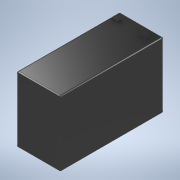
# Autodesk Inventor part: battery
Saved by Autodesk Inventor 2021 (Build 250183000, 183)
## iProperties
Created: 2021-03-02
Part Number: battery
Material: Generic
Document SubType Name: Modeling
Designer: Mateusz
Density: 1 g/cm^3
Appearance: Default
Author: Mateusz
Autodesk Inventor part; units mm, degrees
ref_plane "YZ Plane" through (0, 0, 0) normal (1, 0, 0) x (0, 1, 0)
ref_plane "XZ Plane" through (0, 0, 0) normal (0, 1, 0) x (-1, 0, 0)
ref_plane "XY Plane" through (0, 0, 0) normal (0, 0, 1) x (1, 0, 0)
sketch "Sketch1" plane through (0, 0, 0) normal (0, 1, 0) x (-1, 0, 0)
  line L0 (0, 0) -> (0, -148)
  line L1 (0, -148) -> (63, -148)
  line L2 (63, -148) -> (63, 0)
  line L3 (63, 0) -> (0, 0)
  dimension "d0" = 148
  dimension "d1" = 63
  constraints: 8 end point, 3 perpendicular, 1 vertical
  measures "d0" distance of L0.start L0.end
  measures "d1" distance of L0.end L1.end
extrude "Extrusion1" add sketch "Sketch1" along normal blind 94
sketch "Sketch2" plane through (0, 94, 0) normal (0, 1, 0) x (1, 0, 0)
  line L0 (0, 148) -> (-63, 148) projected
  line L1 (-63, 148) -> (-63, 136)
  line L2 (-63, 148) -> (-63, 0) projected
  line L3 (-63, 136) -> (-55, 136)
  line L4 (-55, 136) -> (-48, 136)
  line L5 (-48, 136) -> (-48, 134)
  line L6 (-48, 134) -> (-55, 134)
  line L7 (-55, 134) -> (-55, 136)
  line L8 (0, 0) -> (0, 148) projected
  line L9 (0, 148) -> (0, 136)
  line L10 (0, 136) -> (-8, 136)
  line L11 (-8, 136) -> (-8, 134)
  line L12 (-8, 134) -> (-15, 134)
  line L13 (-15, 134) -> (-15, 136)
  line L14 (-15, 136) -> (-8, 136)
  dimension "d4" = 12
  dimension "d5" = 8
  dimension "d6" = 7
  dimension "d7" = 2
  dimension "d8" = 12
  dimension "d9" = 8
  dimension "d10" = 2
  dimension "d11" = 7
  constraints: 24 end point, 7 point on line, 5 perpendicular
  measures "d4" distance of L0.end L1.end
  measures "d5" distance of L1.end L3.end
  measures "d6" distance of L3.end L4.end
  measures "d7" distance of L4.end L5.end
  measures "d8" distance of L0.start L9.end
  measures "d9" distance of L9.end L10.end
  measures "d10" distance of L10.end L11.end
  measures "d11" distance of L11.end L12.end
extrude "Extrusion2" add sketch "Sketch2" along normal blind 5
sketch "Sketch3" plane through (-55, 94, -134) normal (0, 0, 1) x (1, 0, 0)
  line L0 (0, 5) -> (7, 5) projected
  line L1 (0, 5) -> (0, 3)
  line L2 (0, 0) -> (0, 5) projected
  line L3 (0, 3) -> (7, 3)
  line L4 (7, 0) -> (7, 5) projected
  line L5 (7, 5) -> (0, 5)
  line L6 (7, 5) -> (7, 3)
  line L7 (40, 5) -> (47, 5) projected
  line L8 (40, 5) -> (47, 5)
  line L9 (47, 5) -> (47, 3)
  line L10 (47, 0) -> (47, 5) projected
  line L11 (47, 3) -> (40, 3)
  line L12 (40, 0) -> (40, 5) projected
  line L13 (40, 5) -> (40, 3)
  point P0 (55, -94)
  dimension "d14" = 2
  dimension "d15" = 2
  constraints: 16 end point, 5 point on line, 2 collinear, 2 perpendicular, 1 parallel
  measures "d14" distance of L0.start L1.end
  measures "d15" distance of L7.end L9.end
extrude "Extrusion3" add sketch "Sketch3" along normal blind 5
fillet "Fillet1" radius 2 12 edges at (0, 94, -74) (-63, 94, -74) (-31.5, 94, -148) (0, 47, -148) (-63, 47, -148) (0, 0, -74) (-31.5, 0, -148) (0, 47, 0) (-31.5, 94, 0) (-63, 47, 0) (-31.5, 0, 0) (-63, 0, -74)
body "Solid1"
